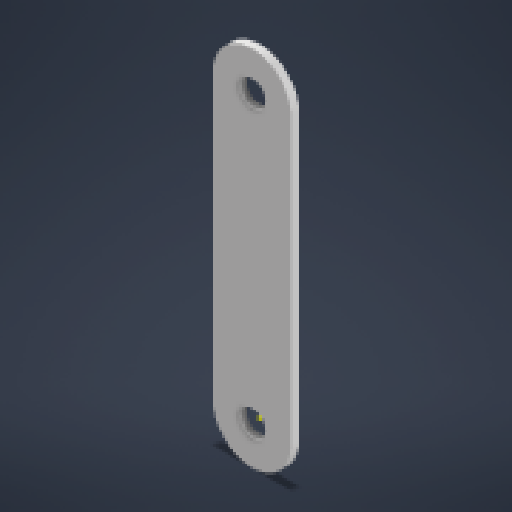
# Autodesk Inventor part: Link3Do
Saved by Autodesk Inventor 2023 (Build 270158000, 158)
## iProperties
Created: 2023-09-10
Part Number: Link3Do
Material: Generic
Document SubType Name: Modeling
Designer: philo
Density: 1 g/cm^3
Appearance: Default
Author: philo
Autodesk Inventor part; units mm, degrees
ref_plane "YZ Plane" through (0, 0, 0) normal (1, 0, 0) x (0, 1, 0)
ref_plane "XZ Plane" through (0, 0, 0) normal (0, 1, 0) x (-1, 0, 0)
ref_plane "XY Plane" through (0, 0, 0) normal (0, 0, 1) x (1, 0, 0)
sketch "Sketch1" plane through (0, 0, 0) normal (0, 0, 1) x (1, 0, 0)
  circle A0 centre (0, 0) radius 5
  circle A1 centre (0, 130) radius 5
  line L0 (-15, 145) -> (15, 145)
  line L1 (15, 145) -> (15, -15)
  line L2 (15, -15) -> (-15, -15)
  line L3 (-15, -15) -> (-15, 145)
  circle A2 centre (0, 130) radius 15
  circle A3 centre (0, 0) radius 15
  point P0 (15, 130)
  point P1 (-15, 130)
  point P2 (-15, 0)
  point P3 (15, 0)
  dimension "d0" = 10
  dimension "d1" = 10
  dimension "d2" = 130
  dimension "d3" = 30
  dimension "d4" = 15
  dimension "d5" = 15
  dimension "d6" = 15
  dimension "d7" = 30
  dimension "d8" = 30
  constraints: 8 end point, 4 centre point, 3 coincident, 2 parallel, 1 horizontal, 1 perpendicular
  measures "d0" diameter of A0
  measures "d1" diameter of A1
  measures "d2" distance of point (0, 0) A1.centre
  measures "d3" distance between parallel lines of L1 L3
  measures "d4" distance from line of point (0, 0) L3
  measures "d5" distance from line of point (0, 0) L2
  measures "d6" distance from line of L0 A1.centre
  measures "d7" diameter of A2
  measures "d8" diameter of A3
sketch "Sketch2" plane through (0, 0, 0) normal (1, 0, 0) x (0, 1, 0)
  point P0 (0, 0)
extrude "Extrusion1" add sketch "Sketch1" along normal blind 3 contours A2 | A2 L1 A3 L3 | A3
sketch "Sketch3" plane through (0, 0, 3) normal (0, 0, 1) x (1, 0, 0)
  circle A0 centre (-10, 97) radius 1.5
  line L0 (-15, 130) -> (-15, 0) projected
  circle A1 centre (0, 130) radius 5 projected
  point P0 (0, 0)
  dimension "d11" = 3
  dimension "d12" = 5
  dimension "d13" = 33
  constraints: 1 centre point
  measures "d11" diameter of A0
  measures "d12" distance from line of L0 A0.centre
  measures "d13" vertical distance of A1.centre A0.centre
extrude "Extrusion2" cut sketch "Sketch3" against normal blind 3 contours A0
body "Solid1"
